Autodesk Fusion 360 part; units mm, degrees
(part 22 of 40)
  line L2950 (-5.2497, -64.1682) -> (-5.2109, -64.3222) construction
  line L2951 (-5.2109, -64.3222) -> (-5.1709, -64.4762) construction
  line L2952 (-5.1709, -64.4762) -> (-5.1297, -64.6301) construction
  line L2953 (-5.1297, -64.6301) -> (-5.0873, -64.7839) construction
  line L2954 (-5.0873, -64.7839) -> (-5.0439, -64.9376) construction
  line L2955 (-5.0439, -64.9376) -> (-4.9993, -65.0912) construction
  line L2956 (-4.9993, -65.0912) -> (-4.9536, -65.2447) construction
  line L2957 (-4.9536, -65.2447) -> (-4.9068, -65.398) construction
  line L2958 (-4.9068, -65.398) -> (-4.8589, -65.5513) construction
  line L2959 (-4.8589, -65.5513) -> (-4.8099, -65.7044) construction
  line L2960 (-4.8099, -65.7044) -> (-4.7599, -65.8574) construction
  line L2961 (-4.7599, -65.8574) -> (-4.7087, -66.0103) construction
  line L2962 (-4.7087, -66.0103) -> (-4.6566, -66.1631) construction
  line L2963 (-4.6566, -66.1631) -> (-4.6035, -66.3158) construction
  line L2964 (-4.6035, -66.3158) -> (-4.5493, -66.4683) construction
  line L2965 (-4.5493, -66.4683) -> (-4.4942, -66.6206) construction
  line L2966 (-4.4942, -66.6206) -> (-4.438, -66.7729) construction
  line L2967 (-4.438, -66.7729) -> (-4.381, -66.925) construction
  line L2968 (-4.381, -66.925) -> (-4.3229, -67.077) construction
  line L2969 (-4.3229, -67.077) -> (-4.2639, -67.2288) construction
  line L2970 (-4.2639, -67.2288) -> (-4.2039, -67.3804) construction
  line L2971 (-4.2039, -67.3804) -> (-4.143, -67.532) construction
  line L2972 (-4.143, -67.532) -> (-4.0812, -67.6833) construction
  line L2973 (-4.0812, -67.6833) -> (-4.0185, -67.8345) construction
  line L2974 (-4.0185, -67.8345) -> (-3.9548, -67.9856) construction
  line L2975 (-3.9548, -67.9856) -> (-3.8903, -68.1365) construction
  line L2976 (-3.8903, -68.1365) -> (-3.8249, -68.2872) construction
  line L2977 (-3.8249, -68.2872) -> (-3.7585, -68.4378) construction
  line L2978 (-3.7585, -68.4378) -> (-3.6913, -68.5882) construction
  line L2979 (-3.6913, -68.5882) -> (-3.6233, -68.7384) construction
  line L2980 (-3.6233, -68.7384) -> (-3.5543, -68.8885) construction
  line L2981 (-3.5543, -68.8885) -> (-3.4846, -69.0384) construction
  line L2982 (-3.4846, -69.0384) -> (-3.4139, -69.1881) construction
  line L2983 (-3.4139, -69.1881) -> (-3.3425, -69.3376) construction
  line L2984 (-3.3425, -69.3376) -> (-3.2701, -69.487) construction
  line L2985 (-3.2701, -69.487) -> (-3.197, -69.6362) construction
  line L2986 (-3.197, -69.6362) -> (-3.123, -69.7852) construction
  line L2987 (-3.123, -69.7852) -> (-3.0482, -69.934) construction
  line L2988 (-3.0482, -69.934) -> (-2.9726, -70.0826) construction
  line L2989 (-2.9726, -70.0826) -> (-2.8962, -70.2311) construction
  line L2990 (-2.8962, -70.2311) -> (-2.819, -70.3793) construction
  line L2991 (-2.819, -70.3793) -> (-2.741, -70.5274) construction
  line L2992 (-2.741, -70.5274) -> (-2.6622, -70.6752) construction
  line L2993 (-2.6622, -70.6752) -> (-2.5826, -70.8229) construction
  line L2994 (-2.5826, -70.8229) -> (-2.5023, -70.9703) construction
  line L2995 (-2.5023, -70.9703) -> (-2.4211, -71.1176) construction
  line L2996 (-2.4211, -71.1176) -> (-2.3556, -71.2352) construction
  line L2997 (-2.3556, -71.2352) -> (-2.3061, -71.3234) construction
  line L2998 (-2.3061, -71.3234) -> (-2.2729, -71.3821) construction
  line L2999 (-2.2729, -71.3821) -> (-2.2563, -71.4115) construction
  line L3000 (-57.9623, 13.005) -> (-59.5542, 13.3622)
  line L3001 (59.1442, 5.5428) -> (60.7685, 5.6951)
  line L3002 (39.2483, -44.5906) -> (40.3263, -45.8153)
  line L3003 (-39.2483, -44.5906) -> (-40.3263, -45.8153)
  line L3004 (5.5428, -59.1442) -> (5.6951, -60.7685)
  spline S40 degree 5 poles (24.1948, 56.0345) (24.2071, 56.0628) (24.2308, 56.1198) (24.264, 56.2062) (24.3039, 56.3229) (24.3478, 56.4711) (24.3873, 56.6208) (24.4241, 56.7714) (24.4595, 56.9226) (24.494, 57.0741) (24.5274, 57.226) (24.5594, 57.3783) (24.5896, 57.5312) (24.6176, 57.6848) (24.6435, 57.8391) (24.6674, 57.994) (24.6897, 58.1494) (24.7105, 58.3052) (24.7301, 58.4614) (24.7485, 58.6179) (24.7658, 58.7747) (24.7818, 58.9318) (24.7965, 59.0893) (24.8098, 59.2471) (24.8218, 59.4053) (24.8325, 59.5638) (24.842, 59.7226) (24.8504, 59.8817) (24.8577, 60.0411) (24.8638, 60.2007) (24.8689, 60.3605) (24.8729, 60.5206) (24.8757, 60.6809) (24.8776, 60.8415) (24.8783, 61.0023) (24.878, 61.1633) (24.8766, 61.3245) (24.8742, 61.4859) (24.8708, 61.6475) (24.8665, 61.8093) (24.8611, 61.9712) (24.8548, 62.1334) (24.8475, 62.2957) (24.8392, 62.4581) (24.83, 62.6207) (24.8199, 62.7835) (24.8088, 62.9464) (24.7967, 63.1095) (24.7838, 63.2727) (24.77, 63.436) (24.7552, 63.5995) (24.7396, 63.7631) (24.723, 63.9268) (24.7056, 64.0906) (24.6873, 64.2545) (24.6681, 64.4185) (24.648, 64.5826) (24.6271, 64.7468) (24.6054, 64.9111) (24.5828, 65.0755) (24.5593, 65.24) (24.535, 65.4046) (24.5098, 65.5692) (24.4839, 65.734) (24.4571, 65.8987) (24.4294, 66.0636) (24.401, 66.2285) (24.3718, 66.3935) (24.3417, 66.5585) (24.3108, 66.7236) (24.2792, 66.8887) (24.2532, 67.0208) (24.2334, 67.1199) (24.22, 67.186) (24.2132, 67.2191) knots 0 0 0 0 0 0 0.01428571 0.02857143 0.04285714 0.05714286 0.07142857 0.08571429 0.1 0.11428571 0.12857143 0.14285714 0.15714286 0.17142857 0.18571429 0.2 0.21428571 0.22857143 0.24285714 0.25714286 0.27142857 0.28571429 0.3 0.31428571 0.32857143 0.34285714 0.35714286 0.37142857 0.38571429 0.4 0.41428571 0.42857143 0.44285714 0.45714286 0.47142857 0.48571429 0.5 0.51428571 0.52857143 0.54285714 0.55714286 0.57142857 0.58571429 0.6 0.61428571 0.62857143 0.64285714 0.65714286 0.67142857 0.68571429 0.7 0.71428571 0.72857143 0.74285714 0.75714286 0.77142857 0.78571429 0.8 0.81428571 0.82857143 0.84285714 0.85714286 0.87142857 0.88571429 0.9 0.91428571 0.92857143 0.94285714 0.95714286 0.97142857 0.98571429 1 1 1 1 1 1
  line L3005 (24.1948, 56.0345) -> (24.2071, 56.0628) construction
  line L3006 (24.2071, 56.0628) -> (24.2308, 56.1198) construction
  line L3007 (24.2308, 56.1198) -> (24.264, 56.2062) construction
  line L3008 (24.264, 56.2062) -> (24.3039, 56.3229) construction
  line L3009 (24.3039, 56.3229) -> (24.3478, 56.4711) construction
  line L3010 (24.3478, 56.4711) -> (24.3873, 56.6208) construction
  line L3011 (24.3873, 56.6208) -> (24.4241, 56.7714) construction
  line L3012 (24.4241, 56.7714) -> (24.4595, 56.9226) construction
  line L3013 (24.4595, 56.9226) -> (24.494, 57.0741) construction
  line L3014 (24.494, 57.0741) -> (24.5274, 57.226) construction
  line L3015 (24.5274, 57.226) -> (24.5594, 57.3783) construction
  line L3016 (24.5594, 57.3783) -> (24.5896, 57.5312) construction
  line L3017 (24.5896, 57.5312) -> (24.6176, 57.6848) construction
  line L3018 (24.6176, 57.6848) -> (24.6435, 57.8391) construction
  line L3019 (24.6435, 57.8391) -> (24.6674, 57.994) construction
  line L3020 (24.6674, 57.994) -> (24.6897, 58.1494) construction
  line L3021 (24.6897, 58.1494) -> (24.7105, 58.3052) construction
  line L3022 (24.7105, 58.3052) -> (24.7301, 58.4614) construction
  line L3023 (24.7301, 58.4614) -> (24.7485, 58.6179) construction
  line L3024 (24.7485, 58.6179) -> (24.7658, 58.7747) construction
  line L3025 (24.7658, 58.7747) -> (24.7818, 58.9318) construction
  line L3026 (24.7818, 58.9318) -> (24.7965, 59.0893) construction
  line L3027 (24.7965, 59.0893) -> (24.8098, 59.2471) construction
  line L3028 (24.8098, 59.2471) -> (24.8218, 59.4053) construction
  line L3029 (24.8218, 59.4053) -> (24.8325, 59.5638) construction
  line L3030 (24.8325, 59.5638) -> (24.842, 59.7226) construction
  line L3031 (24.842, 59.7226) -> (24.8504, 59.8817) construction
  line L3032 (24.8504, 59.8817) -> (24.8577, 60.0411) construction
  line L3033 (24.8577, 60.0411) -> (24.8638, 60.2007) construction
  line L3034 (24.8638, 60.2007) -> (24.8689, 60.3605) construction
  line L3035 (24.8689, 60.3605) -> (24.8729, 60.5206) construction
  line L3036 (24.8729, 60.5206) -> (24.8757, 60.6809) construction
  line L3037 (24.8757, 60.6809) -> (24.8776, 60.8415) construction
  line L3038 (24.8776, 60.8415) -> (24.8783, 61.0023) construction
  line L3039 (24.8783, 61.0023) -> (24.878, 61.1633) construction
  line L3040 (24.878, 61.1633) -> (24.8766, 61.3245) construction
  line L3041 (24.8766, 61.3245) -> (24.8742, 61.4859) construction
  line L3042 (24.8742, 61.4859) -> (24.8708, 61.6475) construction
  line L3043 (24.8708, 61.6475) -> (24.8665, 61.8093) construction
  line L3044 (24.8665, 61.8093) -> (24.8611, 61.9712) construction
  line L3045 (24.8611, 61.9712) -> (24.8548, 62.1334) construction
  line L3046 (24.8548, 62.1334) -> (24.8475, 62.2957) construction
  line L3047 (24.8475, 62.2957) -> (24.8392, 62.4581) construction
  line L3048 (24.8392, 62.4581) -> (24.83, 62.6207) construction
  line L3049 (24.83, 62.6207) -> (24.8199, 62.7835) construction
  line L3050 (24.8199, 62.7835) -> (24.8088, 62.9464) construction
  line L3051 (24.8088, 62.9464) -> (24.7967, 63.1095) construction
  line L3052 (24.7967, 63.1095) -> (24.7838, 63.2727) construction
  line L3053 (24.7838, 63.2727) -> (24.77, 63.436) construction
  line L3054 (24.77, 63.436) -> (24.7552, 63.5995) construction
  line L3055 (24.7552, 63.5995) -> (24.7396, 63.7631) construction
  line L3056 (24.7396, 63.7631) -> (24.723, 63.9268) construction
  line L3057 (24.723, 63.9268) -> (24.7056, 64.0906) construction
  line L3058 (24.7056, 64.0906) -> (24.6873, 64.2545) construction
  line L3059 (24.6873, 64.2545) -> (24.6681, 64.4185) construction
  line L3060 (24.6681, 64.4185) -> (24.648, 64.5826) construction
  line L3061 (24.648, 64.5826) -> (24.6271, 64.7468) construction
  line L3062 (24.6271, 64.7468) -> (24.6054, 64.9111) construction
  line L3063 (24.6054, 64.9111) -> (24.5828, 65.0755) construction
  line L3064 (24.5828, 65.0755) -> (24.5593, 65.24) construction
  line L3065 (24.5593, 65.24) -> (24.535, 65.4046) construction
  line L3066 (24.535, 65.4046) -> (24.5098, 65.5692) construction
  line L3067 (24.5098, 65.5692) -> (24.4839, 65.734) construction
  line L3068 (24.4839, 65.734) -> (24.4571, 65.8987) construction
  line L3069 (24.4571, 65.8987) -> (24.4294, 66.0636) construction
  line L3070 (24.4294, 66.0636) -> (24.401, 66.2285) construction
  line L3071 (24.401, 66.2285) -> (24.3718, 66.3935) construction
  line L3072 (24.3718, 66.3935) -> (24.3417, 66.5585) construction
  line L3073 (24.3417, 66.5585) -> (24.3108, 66.7236) construction
  line L3074 (24.3108, 66.7236) -> (24.2792, 66.8887) construction
  line L3075 (24.2792, 66.8887) -> (24.2532, 67.0208) construction
  line L3076 (24.2532, 67.0208) -> (24.2334, 67.1199) construction
  line L3077 (24.2334, 67.1199) -> (24.22, 67.186) construction
  line L3078 (24.22, 67.186) -> (24.2132, 67.2191) construction
  spline S41 degree 5 poles (13.3622, -59.5542) (13.369, -59.5843) (13.3833, -59.6444) (13.4071, -59.7338) (13.4435, -59.8517) (13.4951, -59.9973) (13.5511, -60.1416) (13.6099, -60.2852) (13.6701, -60.4283) (13.7313, -60.5711) (13.7935, -60.7136) (13.8571, -60.8557) (13.9226, -60.9971) (13.9902, -61.1379) (14.06, -61.2779) (14.1316, -61.4173) (14.205, -61.5561) (14.2797, -61.6944) (14.3557, -61.8322) (14.4327, -61.9697) (14.5109, -62.1067) (14.5904, -62.2432) (14.6711, -62.3792) (14.753, -62.5148) (14.8363, -62.6498) (14.9208, -62.7843) (15.0064, -62.9184) (15.0932, -63.052) (15.181, -63.1852) (15.2698, -63.318) (15.3597, -63.4503) (15.4506, -63.5821) (15.5425, -63.7135) (15.6354, -63.8445) (15.7293, -63.975) (15.8242, -64.105) (15.92, -64.2346) (16.0168, -64.3638) (16.1146, -64.4926) (16.2132, -64.6209) (16.3127, -64.7488) (16.4131, -64.8762) (16.5144, -65.0032) (16.6166, -65.1298) (16.7196, -65.256) (16.8235, -65.3817) (16.9283, -65.507) (17.0338, -65.6318) (17.1402, -65.7562) (17.2474, -65.8802) (17.3555, -66.0038) (17.4643, -66.1269) (17.5739, -66.2497) (17.6842, -66.3719) (17.7954, -66.4938) (17.9073, -66.6152) (18.02, -66.7362) (18.1335, -66.8568) (18.2477, -66.9769) (18.3626, -67.0966) (18.4782, -67.2159) (18.5946, -67.3347) (18.7118, -67.4531) (18.8296, -67.5711) (18.9481, -67.6887) (19.0674, -67.8058) (19.1873, -67.9225) (19.3079, -68.0388) (19.4293, -68.1546) (19.5512, -68.27) (19.6739, -68.385) (19.7726, -68.4767) (19.8469, -68.5452) (19.8966, -68.5908) (19.9215, -68.6136) knots 0 0 0 0 0 0 0.01428571 0.02857143 0.04285714 0.05714286 0.07142857 0.08571429 0.1 0.11428571 0.12857143 0.14285714 0.15714286 0.17142857 0.18571429 0.2 0.21428571 0.22857143 0.24285714 0.25714286 0.27142857 0.28571429 0.3 0.31428571 0.32857143 0.34285714 0.35714286 0.37142857 0.38571429 0.4 0.41428571 0.42857143 0.44285714 0.45714286 0.47142857 0.48571429 0.5 0.51428571 0.52857143 0.54285714 0.55714286 0.57142857 0.58571429 0.6 0.61428571 0.62857143 0.64285714 0.65714286 0.67142857 0.68571429 0.7 0.71428571 0.72857143 0.74285714 0.75714286 0.77142857 0.78571429 0.8 0.81428571 0.82857143 0.84285714 0.85714286 0.87142857 0.88571429 0.9 0.91428571 0.92857143 0.94285714 0.95714286 0.97142857 0.98571429 1 1 1 1 1 1
  line L3079 (13.3622, -59.5542) -> (13.369, -59.5843) construction
  line L3080 (13.369, -59.5843) -> (13.3833, -59.6444) construction
  line L3081 (13.3833, -59.6444) -> (13.4071, -59.7338) construction
  line L3082 (13.4071, -59.7338) -> (13.4435, -59.8517) construction
  line L3083 (13.4435, -59.8517) -> (13.4951, -59.9973) construction
  line L3084 (13.4951, -59.9973) -> (13.5511, -60.1416) construction
  line L3085 (13.5511, -60.1416) -> (13.6099, -60.2852) construction
  line L3086 (13.6099, -60.2852) -> (13.6701, -60.4283) construction
  line L3087 (13.6701, -60.4283) -> (13.7313, -60.5711) construction
  line L3088 (13.7313, -60.5711) -> (13.7935, -60.7136) construction
  line L3089 (13.7935, -60.7136) -> (13.8571, -60.8557) construction
  line L3090 (13.8571, -60.8557) -> (13.9226, -60.9971) construction
  line L3091 (13.9226, -60.9971) -> (13.9902, -61.1379) construction
  line L3092 (13.9902, -61.1379) -> (14.06, -61.2779) construction
  line L3093 (14.06, -61.2779) -> (14.1316, -61.4173) construction
  line L3094 (14.1316, -61.4173) -> (14.205, -61.5561) construction
  line L3095 (14.205, -61.5561) -> (14.2797, -61.6944) construction
  line L3096 (14.2797, -61.6944) -> (14.3557, -61.8322) construction
  line L3097 (14.3557, -61.8322) -> (14.4327, -61.9697) construction
  line L3098 (14.4327, -61.9697) -> (14.5109, -62.1067) construction
  line L3099 (14.5109, -62.1067) -> (14.5904, -62.2432) construction
  line L3100 (14.5904, -62.2432) -> (14.6711, -62.3792) construction
  line L3101 (14.6711, -62.3792) -> (14.753, -62.5148) construction
  line L3102 (14.753, -62.5148) -> (14.8363, -62.6498) construction
  line L3103 (14.8363, -62.6498) -> (14.9208, -62.7843) construction
  line L3104 (14.9208, -62.7843) -> (15.0064, -62.9184) construction
  line L3105 (15.0064, -62.9184) -> (15.0932, -63.052) construction
  line L3106 (15.0932, -63.052) -> (15.181, -63.1852) construction
  line L3107 (15.181, -63.1852) -> (15.2698, -63.318) construction
  line L3108 (15.2698, -63.318) -> (15.3597, -63.4503) construction
  line L3109 (15.3597, -63.4503) -> (15.4506, -63.5821) construction
  line L3110 (15.4506, -63.5821) -> (15.5425, -63.7135) construction
  line L3111 (15.5425, -63.7135) -> (15.6354, -63.8445) construction
  line L3112 (15.6354, -63.8445) -> (15.7293, -63.975) construction
  line L3113 (15.7293, -63.975) -> (15.8242, -64.105) construction
  line L3114 (15.8242, -64.105) -> (15.92, -64.2346) construction
  line L3115 (15.92, -64.2346) -> (16.0168, -64.3638) construction
  line L3116 (16.0168, -64.3638) -> (16.1146, -64.4926) construction
  line L3117 (16.1146, -64.4926) -> (16.2132, -64.6209) construction
  line L3118 (16.2132, -64.6209) -> (16.3127, -64.7488) construction
  line L3119 (16.3127, -64.7488) -> (16.4131, -64.8762) construction
  line L3120 (16.4131, -64.8762) -> (16.5144, -65.0032) construction
  line L3121 (16.5144, -65.0032) -> (16.6166, -65.1298) construction
  line L3122 (16.6166, -65.1298) -> (16.7196, -65.256) construction
  line L3123 (16.7196, -65.256) -> (16.8235, -65.3817) construction
  line L3124 (16.8235, -65.3817) -> (16.9283, -65.507) construction
  line L3125 (16.9283, -65.507) -> (17.0338, -65.6318) construction
  line L3126 (17.0338, -65.6318) -> (17.1402, -65.7562) construction
  line L3127 (17.1402, -65.7562) -> (17.2474, -65.8802) construction
  line L3128 (17.2474, -65.8802) -> (17.3555, -66.0038) construction
  line L3129 (17.3555, -66.0038) -> (17.4643, -66.1269) construction
  line L3130 (17.4643, -66.1269) -> (17.5739, -66.2497) construction
  line L3131 (17.5739, -66.2497) -> (17.6842, -66.3719) construction
  line L3132 (17.6842, -66.3719) -> (17.7954, -66.4938) construction
  line L3133 (17.7954, -66.4938) -> (17.9073, -66.6152) construction
  line L3134 (17.9073, -66.6152) -> (18.02, -66.7362) construction
  line L3135 (18.02, -66.7362) -> (18.1335, -66.8568) construction
  line L3136 (18.1335, -66.8568) -> (18.2477, -66.9769) construction
  line L3137 (18.2477, -66.9769) -> (18.3626, -67.0966) construction
  line L3138 (18.3626, -67.0966) -> (18.4782, -67.2159) construction
  line L3139 (18.4782, -67.2159) -> (18.5946, -67.3347) construction
  line L3140 (18.5946, -67.3347) -> (18.7118, -67.4531) construction
  line L3141 (18.7118, -67.4531) -> (18.8296, -67.5711) construction
  line L3142 (18.8296, -67.5711) -> (18.9481, -67.6887) construction
  line L3143 (18.9481, -67.6887) -> (19.0674, -67.8058) construction
  line L3144 (19.0674, -67.8058) -> (19.1873, -67.9225) construction
  line L3145 (19.1873, -67.9225) -> (19.3079, -68.0388) construction
  line L3146 (19.3079, -68.0388) -> (19.4293, -68.1546) construction
  line L3147 (19.4293, -68.1546) -> (19.5512, -68.27) construction
  line L3148 (19.5512, -68.27) -> (19.6739, -68.385) construction
  line L3149 (19.6739, -68.385) -> (19.7726, -68.4767) construction
  line L3150 (19.7726, -68.4767) -> (19.8469, -68.5452) construction
  line L3151 (19.8469, -68.5452) -> (19.8966, -68.5908) construction
  line L3152 (19.8966, -68.5908) -> (19.9215, -68.6136) construction
  arc A81 (-24.5301, 51.9354) -> (-23.5481, 54.5366) centre (-25.3842, 53.7438) ccw
  spline S42 degree 5 poles (-5.6951, 60.7685) (-5.6979, 60.7993) (-5.7029, 60.8609) (-5.7078, 60.9533) (-5.7097, 61.0766) (-5.7056, 61.231) (-5.6969, 61.3856) (-5.6854, 61.5403) (-5.6723, 61.695) (-5.6583, 61.8498) (-5.6431, 62.0045) (-5.6265, 62.1593) (-5.608, 62.314) (-5.5871, 62.4688) (-5.5641, 62.6235) (-5.539, 62.7782) (-5.5121, 62.9329) (-5.4838, 63.0875) (-5.4542, 63.2421) (-5.4233, 63.3966) (-5.3913, 63.5511) (-5.3579, 63.7055) (-5.3232, 63.8598) (-5.2871, 64.014) (-5.2497, 64.1682) (-5.2109, 64.3222) (-5.1709, 64.4762) (-5.1297, 64.6301) (-5.0873, 64.7839) (-5.0439, 64.9376) (-4.9993, 65.0912) (-4.9536, 65.2447) (-4.9068, 65.398) (-4.8589, 65.5513) (-4.8099, 65.7044) (-4.7599, 65.8574) (-4.7087, 66.0103) (-4.6566, 66.1631) (-4.6035, 66.3158) (-4.5493, 66.4683) (-4.4942, 66.6206) (-4.438, 66.7729) (-4.381, 66.925) (-4.3229, 67.077) (-4.2639, 67.2288) (-4.2039, 67.3804) (-4.143, 67.532) (-4.0812, 67.6833) (-4.0185, 67.8345) (-3.9548, 67.9856) (-3.8903, 68.1365) (-3.8249, 68.2872) (-3.7585, 68.4378) (-3.6913, 68.5882) (-3.6233, 68.7384) (-3.5543, 68.8885) (-3.4846, 69.0384) (-3.4139, 69.1881) (-3.3425, 69.3376) (-3.2701, 69.487) (-3.197, 69.6362) (-3.123, 69.7852) (-3.0482, 69.934) (-2.9726, 70.0826) (-2.8962, 70.2311) (-2.819, 70.3793) (-2.741, 70.5274) (-2.6622, 70.6752) (-2.5826, 70.8229) (-2.5023, 70.9703) (-2.4211, 71.1176) (-2.3556, 71.2352) (-2.3061, 71.3234) (-2.2729, 71.3821) (-2.2563, 71.4115) knots 0 0 0 0 0 0 0.01428571 0.02857143 0.04285714 0.05714286 0.07142857 0.08571429 0.1 0.11428571 0.12857143 0.14285714 0.15714286 0.17142857 0.18571429 0.2 0.21428571 0.22857143 0.24285714 0.25714286 0.27142857 0.28571429 0.3 0.31428571 0.32857143 0.34285714 0.35714286 0.37142857 0.38571429 0.4 0.41428571 0.42857143 0.44285714 0.45714286 0.47142857 0.48571429 0.5 0.51428571 0.52857143 0.54285714 0.55714286 0.57142857 0.58571429 0.6 0.61428571 0.62857143 0.64285714 0.65714286 0.67142857 0.68571429 0.7 0.71428571 0.72857143 0.74285714 0.75714286 0.77142857 0.78571429 0.8 0.81428571 0.82857143 0.84285714 0.85714286 0.87142857 0.88571429 0.9 0.91428571 0.92857143 0.94285714 0.95714286 0.97142857 0.98571429 1 1 1 1 1 1
  line L3153 (-5.6951, 60.7685) -> (-5.6979, 60.7993) construction
  line L3154 (-5.6979, 60.7993) -> (-5.7029, 60.8609) construction
  line L3155 (-5.7029, 60.8609) -> (-5.7078, 60.9533) construction
  line L3156 (-5.7078, 60.9533) -> (-5.7097, 61.0766) construction
  line L3157 (-5.7097, 61.0766) -> (-5.7056, 61.231) construction
  line L3158 (-5.7056, 61.231) -> (-5.6969, 61.3856) construction
  line L3159 (-5.6969, 61.3856) -> (-5.6854, 61.5403) construction
  line L3160 (-5.6854, 61.5403) -> (-5.6723, 61.695) construction
  line L3161 (-5.6723, 61.695) -> (-5.6583, 61.8498) construction
  line L3162 (-5.6583, 61.8498) -> (-5.6431, 62.0045) construction
  line L3163 (-5.6431, 62.0045) -> (-5.6265, 62.1593) construction
  line L3164 (-5.6265, 62.1593) -> (-5.608, 62.314) construction
  line L3165 (-5.608, 62.314) -> (-5.5871, 62.4688) construction
  line L3166 (-5.5871, 62.4688) -> (-5.5641, 62.6235) construction
  line L3167 (-5.5641, 62.6235) -> (-5.539, 62.7782) construction
  line L3168 (-5.539, 62.7782) -> (-5.5121, 62.9329) construction
  line L3169 (-5.5121, 62.9329) -> (-5.4838, 63.0875) construction
  line L3170 (-5.4838, 63.0875) -> (-5.4542, 63.2421) construction
  line L3171 (-5.4542, 63.2421) -> (-5.4233, 63.3966) construction
  line L3172 (-5.4233, 63.3966) -> (-5.3913, 63.5511) construction
  line L3173 (-5.3913, 63.5511) -> (-5.3579, 63.7055) construction
  line L3174 (-5.3579, 63.7055) -> (-5.3232, 63.8598) construction
  line L3175 (-5.3232, 63.8598) -> (-5.2871, 64.014) construction
  line L3176 (-5.2871, 64.014) -> (-5.2497, 64.1682) construction
  line L3177 (-5.2497, 64.1682) -> (-5.2109, 64.3222) construction
  line L3178 (-5.2109, 64.3222) -> (-5.1709, 64.4762) construction
  line L3179 (-5.1709, 64.4762) -> (-5.1297, 64.6301) construction
  line L3180 (-5.1297, 64.6301) -> (-5.0873, 64.7839) construction
  line L3181 (-5.0873, 64.7839) -> (-5.0439, 64.9376) construction
  line L3182 (-5.0439, 64.9376) -> (-4.9993, 65.0912) construction
  line L3183 (-4.9993, 65.0912) -> (-4.9536, 65.2447) construction
  line L3184 (-4.9536, 65.2447) -> (-4.9068, 65.398) construction
  line L3185 (-4.9068, 65.398) -> (-4.8589, 65.5513) construction
  line L3186 (-4.8589, 65.5513) -> (-4.8099, 65.7044) construction
  line L3187 (-4.8099, 65.7044) -> (-4.7599, 65.8574) construction
  line L3188 (-4.7599, 65.8574) -> (-4.7087, 66.0103) construction
  line L3189 (-4.7087, 66.0103) -> (-4.6566, 66.1631) construction
  line L3190 (-4.6566, 66.1631) -> (-4.6035, 66.3158) construction
  line L3191 (-4.6035, 66.3158) -> (-4.5493, 66.4683) construction
  line L3192 (-4.5493, 66.4683) -> (-4.4942, 66.6206) construction
  line L3193 (-4.4942, 66.6206) -> (-4.438, 66.7729) construction
  line L3194 (-4.438, 66.7729) -> (-4.381, 66.925) construction
  line L3195 (-4.381, 66.925) -> (-4.3229, 67.077) construction
  line L3196 (-4.3229, 67.077) -> (-4.2639, 67.2288) construction
  line L3197 (-4.2639, 67.2288) -> (-4.2039, 67.3804) construction
  line L3198 (-4.2039, 67.3804) -> (-4.143, 67.532) construction
  line L3199 (-4.143, 67.532) -> (-4.0812, 67.6833) construction
  line L3200 (-4.0812, 67.6833) -> (-4.0185, 67.8345) construction
  line L3201 (-4.0185, 67.8345) -> (-3.9548, 67.9856) construction
  line L3202 (-3.9548, 67.9856) -> (-3.8903, 68.1365) construction
  line L3203 (-3.8903, 68.1365) -> (-3.8249, 68.2872) construction
  line L3204 (-3.8249, 68.2872) -> (-3.7585, 68.4378) construction
  line L3205 (-3.7585, 68.4378) -> (-3.6913, 68.5882) construction
  line L3206 (-3.6913, 68.5882) -> (-3.6233, 68.7384) construction
  line L3207 (-3.6233, 68.7384) -> (-3.5543, 68.8885) construction
  line L3208 (-3.5543, 68.8885) -> (-3.4846, 69.0384) construction
  line L3209 (-3.4846, 69.0384) -> (-3.4139, 69.1881) construction
  line L3210 (-3.4139, 69.1881) -> (-3.3425, 69.3376) construction
  line L3211 (-3.3425, 69.3376) -> (-3.2701, 69.487) construction
  line L3212 (-3.2701, 69.487) -> (-3.197, 69.6362) construction
  line L3213 (-3.197, 69.6362) -> (-3.123, 69.7852) construction
  line L3214 (-3.123, 69.7852) -> (-3.0482, 69.934) construction
  line L3215 (-3.0482, 69.934) -> (-2.9726, 70.0826) construction
  line L3216 (-2.9726, 70.0826) -> (-2.8962, 70.2311) construction
  line L3217 (-2.8962, 70.2311) -> (-2.819, 70.3793) construction
  line L3218 (-2.819, 70.3793) -> (-2.741, 70.5274) construction
  line L3219 (-2.741, 70.5274) -> (-2.6622, 70.6752) construction
  line L3220 (-2.6622, 70.6752) -> (-2.5826, 70.8229) construction
  line L3221 (-2.5826, 70.8229) -> (-2.5023, 70.9703) construction
  line L3222 (-2.5023, 70.9703) -> (-2.4211, 71.1176) construction
  line L3223 (-2.4211, 71.1176) -> (-2.3556, 71.2352) construction
  line L3224 (-2.3556, 71.2352) -> (-2.3061, 71.3234) construction
  line L3225 (-2.3061, 71.3234) -> (-2.2729, 71.3821) construction
  line L3226 (-2.2729, 71.3821) -> (-2.2563, 71.4115) construction
  arc A82 (-67.2191, 24.2132) -> (-68.6136, 19.9215) centre (0, 0) ccw
  arc A83 (-56.435, 10.6816) -> (-56.9737, 7.2806) centre (0, 0) ccw
  spline S43 degree 5 poles (45.8153, -40.3263) (45.8385, -40.3467) (45.8854, -40.3868) (45.9573, -40.4451) (46.056, -40.5192) (46.1833, -40.6066) (46.3135, -40.6904) (46.4454, -40.772) (46.5782, -40.8524) (46.7117, -40.932) (46.8458, -41.0107) (46.9807, -41.0883) (47.1168, -41.1642) (47.2543, -41.2383) (47.393, -41.3106) (47.5329, -41.3813) (47.6738, -41.4504) (47.8156, -41.5184) (47.9581, -41.5853) (48.1012, -41.6512) (48.245, -41.716) (48.3895, -41.7798) (48.5347, -41.8424) (48.6807, -41.9039) (48.8274, -41.9642) (48.9749, -42.0234) (49.123, -42.0815) (49.2717, -42.1386) (49.421, -42.1947) (49.5709, -42.2499) (49.7214, -42.3041) (49.8724, -42.3574) (50.024, -42.4097) (50.1761, -42.461) (50.3288, -42.5114) (50.482, -42.5608) (50.6358, -42.6094) (50.79, -42.657) (50.9447, -42.7037) (51.0999, -42.7495) (51.2556, -42.7945) (51.4118, -42.8386) (51.5684, -42.8818) (51.7255, -42.9241) (51.883, -42.9656) (52.0409, -43.0063) (52.1993, -43.0461) (52.3581, -43.085) (52.5173, -43.1231) (52.6769, -43.1604) (52.8369, -43.1969) (52.9973, -43.2326) (53.1581, -43.2674) (53.3193, -43.3015) (53.4809, -43.3347) (53.6428, -43.3672) (53.8051, -43.3988) (53.9677, -43.4297) (54.1307, -43.4597) (54.294, -43.489) (54.4577, -43.5175) (54.6217, -43.5453) (54.7861, -43.5723) (54.9508, -43.5984) (55.1158, -43.6239) (55.2811, -43.6486) (55.4467, -43.6725) (55.6126, -43.6956) (55.7789, -43.718) (55.9454, -43.7397) (56.1122, -43.7606) (56.2459, -43.7767) (56.3463, -43.7885) (56.4133, -43.7962) (56.4469, -43.8) knots 0 0 0 0 0 0 0.01428571 0.02857143 0.04285714 0.05714286 0.07142857 0.08571429 0.1 0.11428571 0.12857143 0.14285714 0.15714286 0.17142857 0.18571429 0.2 0.21428571 0.22857143 0.24285714 0.25714286 0.27142857 0.28571429 0.3 0.31428571 0.32857143 0.34285714 0.35714286 0.37142857 0.38571429 0.4 0.41428571 0.42857143 0.44285714 0.45714286 0.47142857 0.48571429 0.5 0.51428571 0.52857143 0.54285714 0.55714286 0.57142857 0.58571429 0.6 0.61428571 0.62857143 0.64285714 0.65714286 0.67142857 0.68571429 0.7 0.71428571 0.72857143 0.74285714 0.75714286 0.77142857 0.78571429 0.8 0.81428571 0.82857143 0.84285714 0.85714286 0.87142857 0.88571429 0.9 0.91428571 0.92857143 0.94285714 0.95714286 0.97142857 0.98571429 1 1 1 1 1 1
  line L3227 (45.8153, -40.3263) -> (45.8385, -40.3467) construction
  line L3228 (45.8385, -40.3467) -> (45.8854, -40.3868) construction
  line L3229 (45.8854, -40.3868) -> (45.9573, -40.4451) construction
  line L3230 (45.9573, -40.4451) -> (46.056, -40.5192) construction
  line L3231 (46.056, -40.5192) -> (46.1833, -40.6066) construction
  line L3232 (46.1833, -40.6066) -> (46.3135, -40.6904) construction
  line L3233 (46.3135, -40.6904) -> (46.4454, -40.772) construction
  line L3234 (46.4454, -40.772) -> (46.5782, -40.8524) construction
  line L3235 (46.5782, -40.8524) -> (46.7117, -40.932) construction
  line L3236 (46.7117, -40.932) -> (46.8458, -41.0107) construction
  line L3237 (46.8458, -41.0107) -> (46.9807, -41.0883) construction
  line L3238 (46.9807, -41.0883) -> (47.1168, -41.1642) construction
  line L3239 (47.1168, -41.1642) -> (47.2543, -41.2383) construction
  line L3240 (47.2543, -41.2383) -> (47.393, -41.3106) construction
  line L3241 (47.393, -41.3106) -> (47.5329, -41.3813) construction
  line L3242 (47.5329, -41.3813) -> (47.6738, -41.4504) construction
  line L3243 (47.6738, -41.4504) -> (47.8156, -41.5184) construction
  line L3244 (47.8156, -41.5184) -> (47.9581, -41.5853) construction
  line L3245 (47.9581, -41.5853) -> (48.1012, -41.6512) construction
  line L3246 (48.1012, -41.6512) -> (48.245, -41.716) construction
  line L3247 (48.245, -41.716) -> (48.3895, -41.7798) construction
  line L3248 (48.3895, -41.7798) -> (48.5347, -41.8424) construction
  line L3249 (48.5347, -41.8424) -> (48.6807, -41.9039) construction
  line L3250 (48.6807, -41.9039) -> (48.8274, -41.9642) construction
  line L3251 (48.8274, -41.9642) -> (48.9749, -42.0234) construction
  line L3252 (48.9749, -42.0234) -> (49.123, -42.0815) construction
  line L3253 (49.123, -42.0815) -> (49.2717, -42.1386) construction
  line L3254 (49.2717, -42.1386) -> (49.421, -42.1947) construction
  line L3255 (49.421, -42.1947) -> (49.5709, -42.2499) construction
  line L3256 (49.5709, -42.2499) -> (49.7214, -42.3041) construction
  line L3257 (49.7214, -42.3041) -> (49.8724, -42.3574) construction
  line L3258 (49.8724, -42.3574) -> (50.024, -42.4097) construction
  line L3259 (50.024, -42.4097) -> (50.1761, -42.461) construction
  line L3260 (50.1761, -42.461) -> (50.3288, -42.5114) construction
  line L3261 (50.3288, -42.5114) -> (50.482, -42.5608) construction
  line L3262 (50.482, -42.5608) -> (50.6358, -42.6094) construction
  line L3263 (50.6358, -42.6094) -> (50.79, -42.657) construction
  line L3264 (50.79, -42.657) -> (50.9447, -42.7037) construction
  line L3265 (50.9447, -42.7037) -> (51.0999, -42.7495) construction
  line L3266 (51.0999, -42.7495) -> (51.2556, -42.7945) construction
  line L3267 (51.2556, -42.7945) -> (51.4118, -42.8386) construction
  line L3268 (51.4118, -42.8386) -> (51.5684, -42.8818) construction
  line L3269 (51.5684, -42.8818) -> (51.7255, -42.9241) construction
  line L3270 (51.7255, -42.9241) -> (51.883, -42.9656) construction
  line L3271 (51.883, -42.9656) -> (52.0409, -43.0063) construction
  line L3272 (52.0409, -43.0063) -> (52.1993, -43.0461) construction
  line L3273 (52.1993, -43.0461) -> (52.3581, -43.085) construction
  line L3274 (52.3581, -43.085) -> (52.5173, -43.1231) construction
  line L3275 (52.5173, -43.1231) -> (52.6769, -43.1604) construction
  line L3276 (52.6769, -43.1604) -> (52.8369, -43.1969) construction
  line L3277 (52.8369, -43.1969) -> (52.9973, -43.2326) construction
  line L3278 (52.9973, -43.2326) -> (53.1581, -43.2674) construction
  line L3279 (53.1581, -43.2674) -> (53.3193, -43.3015) construction
  line L3280 (53.3193, -43.3015) -> (53.4809, -43.3347) construction
  line L3281 (53.4809, -43.3347) -> (53.6428, -43.3672) construction
  line L3282 (53.6428, -43.3672) -> (53.8051, -43.3988) construction
  line L3283 (53.8051, -43.3988) -> (53.9677, -43.4297) construction
  line L3284 (53.9677, -43.4297) -> (54.1307, -43.4597) construction
  line L3285 (54.1307, -43.4597) -> (54.294, -43.489) construction
  line L3286 (54.294, -43.489) -> (54.4577, -43.5175) construction
  line L3287 (54.4577, -43.5175) -> (54.6217, -43.5453) construction
  line L3288 (54.6217, -43.5453) -> (54.7861, -43.5723) construction
  line L3289 (54.7861, -43.5723) -> (54.9508, -43.5984) construction
  line L3290 (54.9508, -43.5984) -> (55.1158, -43.6239) construction
  line L3291 (55.1158, -43.6239) -> (55.2811, -43.6486) construction
  line L3292 (55.2811, -43.6486) -> (55.4467, -43.6725) construction
  line L3293 (55.4467, -43.6725) -> (55.6126, -43.6956) construction
  line L3294 (55.6126, -43.6956) -> (55.7789, -43.718) construction
  line L3295 (55.7789, -43.718) -> (55.9454, -43.7397) construction
  line L3296 (55.9454, -43.7397) -> (56.1122, -43.7606) construction
  line L3297 (56.1122, -43.7606) -> (56.2459, -43.7767) construction
  line L3298 (56.2459, -43.7767) -> (56.3463, -43.7885) construction
  line L3299 (56.3463, -43.7885) -> (56.4133, -43.7962) construction
  line L3300 (56.4133, -43.7962) -> (56.4469, -43.8) construction
  arc A84 (56.4469, -43.8) -> (59.0993, -40.1492) centre (0, 0) ccw
  spline S44 degree 5 poles (-40.3263, -45.8153) (-40.3467, -45.8385) (-40.3868, -45.8854) (-40.4451, -45.9573) (-40.5192, -46.056) (-40.6066, -46.1833) (-40.6904, -46.3135) (-40.772, -46.4454) (-40.8524, -46.5782) (-40.932, -46.7117) (-41.0107, -46.8458) (-41.0883, -46.9807) (-41.1642, -47.1168) (-41.2383, -47.2543) (-41.3106, -47.393) (-41.3813, -47.5329) (-41.4504, -47.6738) (-41.5184, -47.8156) (-41.5853, -47.9581) (-41.6512, -48.1012) (-41.716, -48.245) (-41.7798, -48.3895) (-41.8424, -48.5347) (-41.9039, -48.6807) (-41.9642, -48.8274) (-42.0234, -48.9749) (-42.0815, -49.123) (-42.1386, -49.2717) (-42.1947, -49.421) (-42.2499, -49.5709) (-42.3041, -49.7214) (-42.3574, -49.8724) (-42.4097, -50.024) (-42.461, -50.1761) (-42.5114, -50.3288) (-42.5608, -50.482) (-42.6094, -50.6358) (-42.657, -50.79) (-42.7037, -50.9447) (-42.7495, -51.0999) (-42.7945, -51.2556) (-42.8386, -51.4118) (-42.8818, -51.5684) (-42.9241, -51.7255) (-42.9656, -51.883) (-43.0063, -52.0409) (-43.0461, -52.1993) (-43.085, -52.3581) (-43.1231, -52.5173) (-43.1604, -52.6769) (-43.1969, -52.8369) (-43.2326, -52.9973) (-43.2674, -53.1581) (-43.3015, -53.3193) (-43.3347, -53.4809) (-43.3672, -53.6428) (-43.3988, -53.8051) (-43.4297, -53.9677) (-43.4597, -54.1307) (-43.489, -54.294) (-43.5175, -54.4577) (-43.5453, -54.6217) (-43.5723, -54.7861) (-43.5984, -54.9508) (-43.6239, -55.1158) (-43.6486, -55.2811) (-43.6725, -55.4467) (-43.6956, -55.6126) (-43.718, -55.7789) (-43.7397, -55.9454) (-43.7606, -56.1122) (-43.7767, -56.2459) (-43.7885, -56.3463) (-43.7962, -56.4133) (-43.8, -56.4469) knots 0 0 0 0 0 0 0.01428571 0.02857143 0.04285714 0.05714286 0.07142857 0.08571429 0.1 0.11428571 0.12857143 0.14285714 0.15714286 0.17142857 0.18571429 0.2 0.21428571 0.22857143 0.24285714 0.25714286 0.27142857 0.28571429 0.3 0.31428571 0.32857143 0.34285714 0.35714286 0.37142857 0.38571429 0.4 0.41428571 0.42857143 0.44285714 0.45714286 0.47142857 0.48571429 0.5 0.51428571 0.52857143 0.54285714 0.55714286 0.57142857 0.58571429 0.6 0.61428571 0.62857143 0.64285714 0.65714286 0.67142857 0.68571429 0.7 0.71428571 0.72857143 0.74285714 0.75714286 0.77142857 0.78571429 0.8 0.81428571 0.82857143 0.84285714 0.85714286 0.87142857 0.88571429 0.9 0.91428571 0.92857143 0.94285714 0.95714286 0.97142857 0.98571429 1 1 1 1 1 1
  line L3301 (-40.3263, -45.8153) -> (-40.3467, -45.8385) construction
  line L3302 (-40.3467, -45.8385) -> (-40.3868, -45.8854) construction
  line L3303 (-40.3868, -45.8854) -> (-40.4451, -45.9573) construction
  line L3304 (-40.4451, -45.9573) -> (-40.5192, -46.056) construction
  line L3305 (-40.5192, -46.056) -> (-40.6066, -46.1833) construction
  line L3306 (-40.6066, -46.1833) -> (-40.6904, -46.3135) construction
  line L3307 (-40.6904, -46.3135) -> (-40.772, -46.4454) construction
  line L3308 (-40.772, -46.4454) -> (-40.8524, -46.5782) construction
  line L3309 (-40.8524, -46.5782) -> (-40.932, -46.7117) construction
  line L3310 (-40.932, -46.7117) -> (-41.0107, -46.8458) construction
  line L3311 (-41.0107, -46.8458) -> (-41.0883, -46.9807) construction
  line L3312 (-41.0883, -46.9807) -> (-41.1642, -47.1168) construction
  line L3313 (-41.1642, -47.1168) -> (-41.2383, -47.2543) construction
  line L3314 (-41.2383, -47.2543) -> (-41.3106, -47.393) construction
  line L3315 (-41.3106, -47.393) -> (-41.3813, -47.5329) construction
  line L3316 (-41.3813, -47.5329) -> (-41.4504, -47.6738) construction
  line L3317 (-41.4504, -47.6738) -> (-41.5184, -47.8156) construction
  line L3318 (-41.5184, -47.8156) -> (-41.5853, -47.9581) construction
  line L3319 (-41.5853, -47.9581) -> (-41.6512, -48.1012) construction
  line L3320 (-41.6512, -48.1012) -> (-41.716, -48.245) construction
  line L3321 (-41.716, -48.245) -> (-41.7798, -48.3895) construction
  line L3322 (-41.7798, -48.3895) -> (-41.8424, -48.5347) construction
  line L3323 (-41.8424, -48.5347) -> (-41.9039, -48.6807) construction
  line L3324 (-41.9039, -48.6807) -> (-41.9642, -48.8274) construction
  line L3325 (-41.9642, -48.8274) -> (-42.0234, -48.9749) construction
  line L3326 (-42.0234, -48.9749) -> (-42.0815, -49.123) construction
  line L3327 (-42.0815, -49.123) -> (-42.1386, -49.2717) construction
  line L3328 (-42.1386, -49.2717) -> (-42.1947, -49.421) construction
  line L3329 (-42.1947, -49.421) -> (-42.2499, -49.5709) construction
  line L3330 (-42.2499, -49.5709) -> (-42.3041, -49.7214) construction
  line L3331 (-42.3041, -49.7214) -> (-42.3574, -49.8724) construction
  line L3332 (-42.3574, -49.8724) -> (-42.4097, -50.024) construction
  line L3333 (-42.4097, -50.024) -> (-42.461, -50.1761) construction
  line L3334 (-42.461, -50.1761) -> (-42.5114, -50.3288) construction
  line L3335 (-42.5114, -50.3288) -> (-42.5608, -50.482) construction
  line L3336 (-42.5608, -50.482) -> (-42.6094, -50.6358) construction
  line L3337 (-42.6094, -50.6358) -> (-42.657, -50.79) construction
  line L3338 (-42.657, -50.79) -> (-42.7037, -50.9447) construction
  line L3339 (-42.7037, -50.9447) -> (-42.7495, -51.0999) construction
  line L3340 (-42.7495, -51.0999) -> (-42.7945, -51.2556) construction
  line L3341 (-42.7945, -51.2556) -> (-42.8386, -51.4118) construction
  line L3342 (-42.8386, -51.4118) -> (-42.8818, -51.5684) construction
  line L3343 (-42.8818, -51.5684) -> (-42.9241, -51.7255) construction
  line L3344 (-42.9241, -51.7255) -> (-42.9656, -51.883) construction
  line L3345 (-42.9656, -51.883) -> (-43.0063, -52.0409) construction
  line L3346 (-43.0063, -52.0409) -> (-43.0461, -52.1993) construction
  line L3347 (-43.0461, -52.1993) -> (-43.085, -52.3581) construction
  line L3348 (-43.085, -52.3581) -> (-43.1231, -52.5173) construction
  line L3349 (-43.1231, -52.5173) -> (-43.1604, -52.6769) construction
  line L3350 (-43.1604, -52.6769) -> (-43.1969, -52.8369) construction
  line L3351 (-43.1969, -52.8369) -> (-43.2326, -52.9973) construction
  line L3352 (-43.2326, -52.9973) -> (-43.2674, -53.1581) construction
  line L3353 (-43.2674, -53.1581) -> (-43.3015, -53.3193) construction
  line L3354 (-43.3015, -53.3193) -> (-43.3347, -53.4809) construction
  line L3355 (-43.3347, -53.4809) -> (-43.3672, -53.6428) construction
  line L3356 (-43.3672, -53.6428) -> (-43.3988, -53.8051) construction
  line L3357 (-43.3988, -53.8051) -> (-43.4297, -53.9677) construction
  line L3358 (-43.4297, -53.9677) -> (-43.4597, -54.1307) construction
  line L3359 (-43.4597, -54.1307) -> (-43.489, -54.294) construction
  line L3360 (-43.489, -54.294) -> (-43.5175, -54.4577) construction
  line L3361 (-43.5175, -54.4577) -> (-43.5453, -54.6217) construction
  line L3362 (-43.5453, -54.6217) -> (-43.5723, -54.7861) construction
  line L3363 (-43.5723, -54.7861) -> (-43.5984, -54.9508) construction
  line L3364 (-43.5984, -54.9508) -> (-43.6239, -55.1158) construction
  line L3365 (-43.6239, -55.1158) -> (-43.6486, -55.2811) construction
  line L3366 (-43.6486, -55.2811) -> (-43.6725, -55.4467) construction
  line L3367 (-43.6725, -55.4467) -> (-43.6956, -55.6126) construction
  line L3368 (-43.6956, -55.6126) -> (-43.718, -55.7789) construction
  line L3369 (-43.718, -55.7789) -> (-43.7397, -55.9454) construction
  line L3370 (-43.7397, -55.9454) -> (-43.7606, -56.1122) construction
  line L3371 (-43.7606, -56.1122) -> (-43.7767, -56.2459) construction
  line L3372 (-43.7767, -56.2459) -> (-43.7885, -56.3463) construction
  line L3373 (-43.7885, -56.3463) -> (-43.7962, -56.4133) construction
  line L3374 (-43.7962, -56.4133) -> (-43.8, -56.4469) construction
  arc A85 (-68.6136, -19.9215) -> (-67.2191, -24.2132) centre (0, 0) ccw
  arc A86 (50.3721, -27.5982) -> (51.1066, -30.2798) centre (52.1261, -28.5592) ccw
  spline S45 degree 5 poles (-59.5542, 13.3622) (-59.5843, 13.369) (-59.6444, 13.3833) (-59.7338, 13.4071) (-59.8517, 13.4435) (-59.9973, 13.4951) (-60.1416, 13.5511) (-60.2852, 13.6099) (-60.4283, 13.6701) (-60.5711, 13.7313) (-60.7136, 13.7935) (-60.8557, 13.8571) (-60.9971, 13.9226) (-61.1379, 13.9902) (-61.2779, 14.06) (-61.4173, 14.1316) (-61.5561, 14.205) (-61.6944, 14.2797) (-61.8322, 14.3557) (-61.9697, 14.4327) (-62.1067, 14.5109) (-62.2432, 14.5904) (-62.3792, 14.6711) (-62.5148, 14.753) (-62.6498, 14.8363) (-62.7843, 14.9208) (-62.9184, 15.0064) (-63.052, 15.0932) (-63.1852, 15.181) (-63.318, 15.2698) (-63.4503, 15.3597) (-63.5821, 15.4506) (-63.7135, 15.5425) (-63.8445, 15.6354) (-63.975, 15.7293) (-64.105, 15.8242) (-64.2346, 15.92) (-64.3638, 16.0168) (-64.4926, 16.1146) (-64.6209, 16.2132) (-64.7488, 16.3127) (-64.8762, 16.4131) (-65.0032, 16.5144) (-65.1298, 16.6166) (-65.256, 16.7196) (-65.3817, 16.8235) (-65.507, 16.9283) (-65.6318, 17.0338) (-65.7562, 17.1402) (-65.8802, 17.2474) (-66.0038, 17.3555) (-66.1269, 17.4643) (-66.2497, 17.5739) (-66.3719, 17.6842) (-66.4938, 17.7954) (-66.6152, 17.9073) (-66.7362, 18.02) (-66.8568, 18.1335) (-66.9769, 18.2477) (-67.0966, 18.3626) (-67.2159, 18.4782) (-67.3347, 18.5946) (-67.4531, 18.7118) (-67.5711, 18.8296) (-67.6887, 18.9481) (-67.8058, 19.0674) (-67.9225, 19.1873) (-68.0388, 19.3079) (-68.1546, 19.4293) (-68.27, 19.5512) (-68.385, 19.6739) (-68.4767, 19.7726) (-68.5452, 19.8469) (-68.5908, 19.8966) (-68.6136, 19.9215) knots 0 0 0 0 0 0 0.01428571 0.02857143 0.04285714 0.05714286 0.07142857 0.08571429 0.1 0.11428571 0.12857143 0.14285714 0.15714286 0.17142857 0.18571429 0.2 0.21428571 0.22857143 0.24285714 0.25714286 0.27142857 0.28571429 0.3 0.31428571 0.32857143 0.34285714 0.35714286 0.37142857 0.38571429 0.4 0.41428571 0.42857143 0.44285714 0.45714286 0.47142857 0.48571429 0.5 0.51428571 0.52857143 0.54285714 0.55714286 0.57142857 0.58571429 0.6 0.61428571 0.62857143 0.64285714 0.65714286 0.67142857 0.68571429 0.7 0.71428571 0.72857143 0.74285714 0.75714286 0.77142857 0.78571429 0.8 0.81428571 0.82857143 0.84285714 0.85714286 0.87142857 0.88571429 0.9 0.91428571 0.92857143 0.94285714 0.95714286 0.97142857 0.98571429 1 1 1 1 1 1
  line L3375 (-59.5542, 13.3622) -> (-59.5843, 13.369) construction
  line L3376 (-59.5843, 13.369) -> (-59.6444, 13.3833) construction
  line L3377 (-59.6444, 13.3833) -> (-59.7338, 13.4071) construction
  line L3378 (-59.7338, 13.4071) -> (-59.8517, 13.4435) construction
  line L3379 (-59.8517, 13.4435) -> (-59.9973, 13.4951) construction
  line L3380 (-59.9973, 13.4951) -> (-60.1416, 13.5511) construction
  line L3381 (-60.1416, 13.5511) -> (-60.2852, 13.6099) construction
  line L3382 (-60.2852, 13.6099) -> (-60.4283, 13.6701) construction
  line L3383 (-60.4283, 13.6701) -> (-60.5711, 13.7313) construction
  line L3384 (-60.5711, 13.7313) -> (-60.7136, 13.7935) construction
  line L3385 (-60.7136, 13.7935) -> (-60.8557, 13.8571) construction
  line L3386 (-60.8557, 13.8571) -> (-60.9971, 13.9226) construction
  line L3387 (-60.9971, 13.9226) -> (-61.1379, 13.9902) construction
  line L3388 (-61.1379, 13.9902) -> (-61.2779, 14.06) construction
  line L3389 (-61.2779, 14.06) -> (-61.4173, 14.1316) construction
  line L3390 (-61.4173, 14.1316) -> (-61.5561, 14.205) construction
  line L3391 (-61.5561, 14.205) -> (-61.6944, 14.2797) construction
  line L3392 (-61.6944, 14.2797) -> (-61.8322, 14.3557) construction
  line L3393 (-61.8322, 14.3557) -> (-61.9697, 14.4327) construction
  line L3394 (-61.9697, 14.4327) -> (-62.1067, 14.5109) construction
  line L3395 (-62.1067, 14.5109) -> (-62.2432, 14.5904) construction
  line L3396 (-62.2432, 14.5904) -> (-62.3792, 14.6711) construction
  line L3397 (-62.3792, 14.6711) -> (-62.5148, 14.753) construction
  line L3398 (-62.5148, 14.753) -> (-62.6498, 14.8363) construction
  line L3399 (-62.6498, 14.8363) -> (-62.7843, 14.9208) construction
  line L3400 (-62.7843, 14.9208) -> (-62.9184, 15.0064) construction
  line L3401 (-62.9184, 15.0064) -> (-63.052, 15.0932) construction
  line L3402 (-63.052, 15.0932) -> (-63.1852, 15.181) construction
  line L3403 (-63.1852, 15.181) -> (-63.318, 15.2698) construction
  line L3404 (-63.318, 15.2698) -> (-63.4503, 15.3597) construction
  line L3405 (-63.4503, 15.3597) -> (-63.5821, 15.4506) construction
  line L3406 (-63.5821, 15.4506) -> (-63.7135, 15.5425) construction
  line L3407 (-63.7135, 15.5425) -> (-63.8445, 15.6354) construction
  line L3408 (-63.8445, 15.6354) -> (-63.975, 15.7293) construction
  line L3409 (-63.975, 15.7293) -> (-64.105, 15.8242) construction
  line L3410 (-64.105, 15.8242) -> (-64.2346, 15.92) construction
  line L3411 (-64.2346, 15.92) -> (-64.3638, 16.0168) construction
  line L3412 (-64.3638, 16.0168) -> (-64.4926, 16.1146) construction
  line L3413 (-64.4926, 16.1146) -> (-64.6209, 16.2132) construction
  line L3414 (-64.6209, 16.2132) -> (-64.7488, 16.3127) construction
  line L3415 (-64.7488, 16.3127) -> (-64.8762, 16.4131) construction
  line L3416 (-64.8762, 16.4131) -> (-65.0032, 16.5144) construction
  line L3417 (-65.0032, 16.5144) -> (-65.1298, 16.6166) construction
  line L3418 (-65.1298, 16.6166) -> (-65.256, 16.7196) construction
  line L3419 (-65.256, 16.7196) -> (-65.3817, 16.8235) construction
  line L3420 (-65.3817, 16.8235) -> (-65.507, 16.9283) construction
  line L3421 (-65.507, 16.9283) -> (-65.6318, 17.0338) construction
  line L3422 (-65.6318, 17.0338) -> (-65.7562, 17.1402) construction
  line L3423 (-65.7562, 17.1402) -> (-65.8802, 17.2474) construction
  line L3424 (-65.8802, 17.2474) -> (-66.0038, 17.3555) construction
  line L3425 (-66.0038, 17.3555) -> (-66.1269, 17.4643) construction
  line L3426 (-66.1269, 17.4643) -> (-66.2497, 17.5739) construction
  line L3427 (-66.2497, 17.5739) -> (-66.3719, 17.6842) construction
  line L3428 (-66.3719, 17.6842) -> (-66.4938, 17.7954) construction
  line L3429 (-66.4938, 17.7954) -> (-66.6152, 17.9073) construction
  line L3430 (-66.6152, 17.9073) -> (-66.7362, 18.02) construction
  line L3431 (-66.7362, 18.02) -> (-66.8568, 18.1335) construction
  line L3432 (-66.8568, 18.1335) -> (-66.9769, 18.2477) construction
  line L3433 (-66.9769, 18.2477) -> (-67.0966, 18.3626) construction
  line L3434 (-67.0966, 18.3626) -> (-67.2159, 18.4782) construction
  line L3435 (-67.2159, 18.4782) -> (-67.3347, 18.5946) construction
  line L3436 (-67.3347, 18.5946) -> (-67.4531, 18.7118) construction
  line L3437 (-67.4531, 18.7118) -> (-67.5711, 18.8296) construction
  line L3438 (-67.5711, 18.8296) -> (-67.6887, 18.9481) construction
  line L3439 (-67.6887, 18.9481) -> (-67.8058, 19.0674) construction
  line L3440 (-67.8058, 19.0674) -> (-67.9225, 19.1873) construction
  line L3441 (-67.9225, 19.1873) -> (-68.0388, 19.3079) construction
  line L3442 (-68.0388, 19.3079) -> (-68.1546, 19.4293) construction
  line L3443 (-68.1546, 19.4293) -> (-68.27, 19.5512) construction
  line L3444 (-68.27, 19.5512) -> (-68.385, 19.6739) construction
  line L3445 (-68.385, 19.6739) -> (-68.4767, 19.7726) construction
  line L3446 (-68.4767, 19.7726) -> (-68.5452, 19.8469) construction
  line L3447 (-68.5452, 19.8469) -> (-68.5908, 19.8966) construction
  line L3448 (-68.5908, 19.8966) -> (-68.6136, 19.9215) construction
  spline S46 degree 5 poles (13.3622, 59.5542) (13.369, 59.5843) (13.3833, 59.6444) (13.4071, 59.7338) (13.4435, 59.8517) (13.4951, 59.9973) (13.5511, 60.1416) (13.6099, 60.2852) (13.6701, 60.4283) (13.7313, 60.5711) (13.7935, 60.7136) (13.8571, 60.8557) (13.9226, 60.9971) (13.9902, 61.1379) (14.06, 61.2779) (14.1316, 61.4173) (14.205, 61.5561) (14.2797, 61.6944) (14.3557, 61.8322) (14.4327, 61.9697) (14.5109, 62.1067) (14.5904, 62.2432) (14.6711, 62.3792) (14.753, 62.5148) (14.8363, 62.6498) (14.9208, 62.7843) (15.0064, 62.9184) (15.0932, 63.052) (15.181, 63.1852) (15.2698, 63.318) (15.3597, 63.4503) (15.4506, 63.5821) (15.5425, 63.7135) (15.6354, 63.8445) (15.7293, 63.975) (15.8242, 64.105) (15.92, 64.2346) (16.0168, 64.3638) (16.1146, 64.4926) (16.2132, 64.6209) (16.3127, 64.7488) (16.4131, 64.8762) (16.5144, 65.0032) (16.6166, 65.1298) (16.7196, 65.256) (16.8235, 65.3817) (16.9283, 65.507) (17.0338, 65.6318) (17.1402, 65.7562) (17.2474, 65.8802) (17.3555, 66.0038) (17.4643, 66.1269) (17.5739, 66.2497) (17.6842, 66.3719) (17.7954, 66.4938) (17.9073, 66.6152) (18.02, 66.7362) (18.1335, 66.8568) (18.2477, 66.9769) (18.3626, 67.0966) (18.4782, 67.2159) (18.5946, 67.3347) (18.7118, 67.4531) (18.8296, 67.5711) (18.9481, 67.6887) (19.0674, 67.8058) (19.1873, 67.9225) (19.3079, 68.0388) (19.4293, 68.1546) (19.5512, 68.27) (19.6739, 68.385) (19.7726, 68.4767) (19.8469, 68.5452) (19.8966, 68.5908) (19.9215, 68.6136) knots 0 0 0 0 0 0 0.01428571 0.02857143 0.04285714 0.05714286 0.07142857 0.08571429 0.1 0.11428571 0.12857143 0.14285714 0.15714286 0.17142857 0.18571429 0.2 0.21428571 0.22857143 0.24285714 0.25714286 0.27142857 0.28571429 0.3 0.31428571 0.32857143 0.34285714 0.35714286 0.37142857 0.38571429 0.4 0.41428571 0.42857143 0.44285714 0.45714286 0.47142857 0.48571429 0.5 0.51428571 0.52857143 0.54285714 0.55714286 0.57142857 0.58571429 0.6 0.61428571 0.62857143 0.64285714 0.65714286 0.67142857 0.68571429 0.7 0.71428571 0.72857143 0.74285714 0.75714286 0.77142857 0.78571429 0.8 0.81428571 0.82857143 0.84285714 0.85714286 0.87142857 0.88571429 0.9 0.91428571 0.92857143 0.94285714 0.95714286 0.97142857 0.98571429 1 1 1 1 1 1